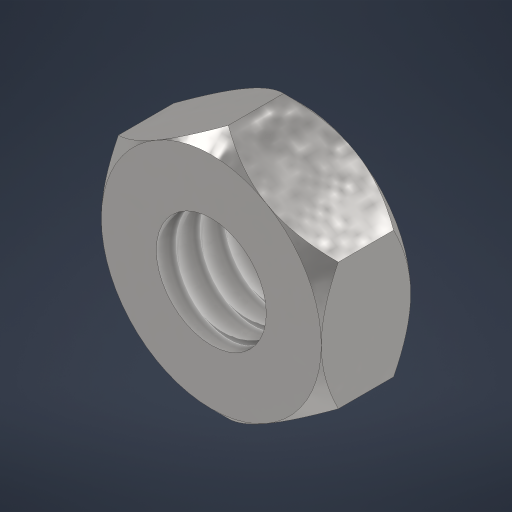
# Autodesk Inventor part: M1.6
Saved by Autodesk Inventor 2023.1 (Build 271208000, 208)
## iProperties
Created: 2022-08-21
Part Number: M1.6
Material: Steel, Galvanized
Document SubType Name: Modeling
Designer: ABL
Density: 7.85 g/cm^3
Appearance: Galvanized
Author: ABL
Autodesk Inventor part; units mm, degrees
ref_plane "YZ Plane" through (0, 0, 0) normal (1, 0, 0) x (0, 1, 0)
ref_plane "XZ Plane" through (0, 0, 0) normal (0, 1, 0) x (-1, 0, 0)
ref_plane "XY Plane" through (0, 0, 0) normal (0, 0, 1) x (1, 0, 0)
sketch "Sketch1" plane through (0, 0, 0) normal (0, 0, 1) x (1, 0, 0)
  line L0 (0, 1.8475) -> (1.6, 0.9238)
  line L1 (1.6, 0.9238) -> (1.6, -0.9238)
  line L2 (1.6, -0.9238) -> (0, -1.8475)
  line L3 (0, -1.8475) -> (-1.6, -0.9238)
  line L4 (-1.6, -0.9238) -> (-1.6, 0.9238)
  line L5 (-1.6, 0.9238) -> (0, 1.8475)
  point P0 (0, 0)
  point P1 (0, 0)
  dimension "d0" = 3.2
  constraints: 12 end point, 1 coincident, 1 vertical, 13 other
  measures "d0" distance between parallel lines of L1 L4
extrude "Main Body" add sketch "Sketch1" along normal blind 1.3
sketch "Sketch2" plane through (0, 0, 1.3) normal (0, 0, 1) x (1, 0, 0)
  circle A0 centre (0, 0) radius 1.6
  line L0 (1.6, -0.9238) -> (1.6, 0.9238) construction
  point P0 (1.6, 0)
  constraints: 1 coincident, 1 horizontal alignment, 1 midpoint, 2 other
extrude "Front Taper" cut sketch "Sketch2" against normal up to surface (1.3 mm away) draft 45 keep common part
sketch "Sketch3" plane through (0, 0, 0) normal (0, 0, -1) x (-1, 0, 0)
  circle A0 centre (0, 0) radius 1.6
  line L0 (-1.6, -0.9238) -> (-1.6, 0.9238) projected
  point P0 (-1.6, 0)
  constraints: 1 coincident, 1 horizontal alignment, 1 midpoint, 2 other
extrude "Back Taper" cut sketch "Sketch3" against normal up to surface (1.3 mm away) draft 45 keep common part
sketch "Sketch4" plane through (0, 0, 1.3) normal (0, 0, 1) x (1, 0, 0)
  circle A0 centre (0, 0) radius 0.8
  dimension "d9" = 1.6
  constraints: 1 centre point, 1 coincident
  measures "d9" diameter of A0
extrude "Center Hole" cut sketch "Sketch4" against normal up to surface (1.3 mm away)
thread "Thread1" size "M1.6x0.35" class "6H" standard "ANSI Metric M Profile" full length
sketch "Sketch5" plane through (0, 0, 0) normal (1, 0, 0) x (0, 1, 0)
  line L0 (-1.0281, 1.9183) -> (-0.8, 2.05)
  line L1 (-0.8, 2.05) -> (-0.8, 1.7)
  line L2 (-0.8, 1.7) -> (-1.0281, 1.8317)
  line L3 (-1.1031, 1.875) -> (-0.8, 1.875) construction
  line L4 (-0.8, 1.3) -> (0.8, 1.3) construction
  arc A0 (-1.0281, 1.9183) -> (-1.0281, 1.8317) centre (-1.0031, 1.875) ccw
  point P0 (0, 0)
  point P1 (-0.901, 1.875)
  dimension "d14" = 0.35
  dimension "d15" = 0.4
  dimension "d16" = 0
  dimension "d17" = 0.05
  constraints: 8 end point, 2 point on circle, 2 point on line, 2 tangent, 1 centre point, 1 horizontal, 1 midpoint, 7 other
  measures "d14" distance of L0.end L1.end
  measures "d15" distance from line of L4 L1.end
  measures "d16" distance from line of L4.start L1
  measures "d17" radius of A0
coil "Coil1" [suppressed]
equation "\"d0\" = size"
equation "\"d1\" = thickness"
equation "\"d9\" = nominalDiameter"
equation "\"d14\" = threadPitch"
equation "\"d15\" = 1.14286 * threadPitch"
equation "\"d17\" = 0.142857 * threadPitch"
equation "\"d18\" = threadPitch"
equation "\"d19\" = 1.57143 * thickness"
equation "\"size\" = 3.2"
equation "\"thickness\" = 1.3"
equation "\"nominalDiameter\" = 1.6"
equation "\"threadPitch\" = 0.35"
body "Solid1"
